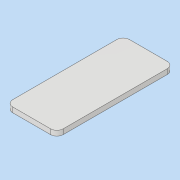
# Autodesk Inventor part: HallEffectSensorCaseLid
Saved by Autodesk Inventor 2017 (Build 210142000, 142)
## iProperties
Created: 2018-04-11
Part Number: HallEffectSensorCaseLid
Material: ABS Plastic
Document SubType Name: Modeling
Designer: Derek Wider
Density: 1.06 g/cm^3
Appearance: Smooth - White
Author: Derek Wider
Autodesk Inventor part; units mm, degrees
ref_plane "YZ Plane" through (0, 0, 0) normal (1, 0, 0) x (0, 1, 0)
ref_plane "XZ Plane" through (0, 0, 0) normal (0, 1, 0) x (-1, 0, 0)
ref_plane "XY Plane" through (0, 0, 0) normal (0, 0, 1) x (1, 0, 0)
sketch "Sketch1" plane through (0, 0, 0) normal (0, 1, 0) x (-1, 0, 0)
  line L0 (0, 0) -> (10.16, 0)
  line L1 (10.16, 0) -> (10.16, -23.495)
  line L2 (10.16, -23.495) -> (0, -23.495)
  line L3 (0, -23.495) -> (0, 0)
  line L4 (8.001, -21.336) -> (8.001, -2.159)
  line L5 (8.001, -2.159) -> (2.159, -2.159)
  line L6 (2.159, -2.159) -> (2.159, -21.336)
  line L7 (2.159, -21.336) -> (8.001, -21.336)
  dimension "d0" = 23.495
  dimension "d1" = 10.16
  dimension "d2" = 2.159
  constraints: 16 end point, 4 parallel, 2 perpendicular, 1 horizontal, 3 other
  measures "d0" distance of L0.end L1.end
  measures "d1" distance of L0.start L0.end
  measures "d2" distance between parallel lines of L1 L4
extrude "Extrusion1" add sketch "Sketch1" along normal blind 1.016 contours L0 L1 L2 L3 | L7 L6 L5 L4
extrude "Extrusion2" add sketch "Sketch1" against normal blind 1.016 contours L7 L6 L5 L4
fillet "Fillet1" radius 1.27 4 edges at (0, 0.508, 0) (0, 0.508, -23.495) (-10.16, 0.508, -23.495) (-10.16, 0.508, 0)
body "Solid1"
